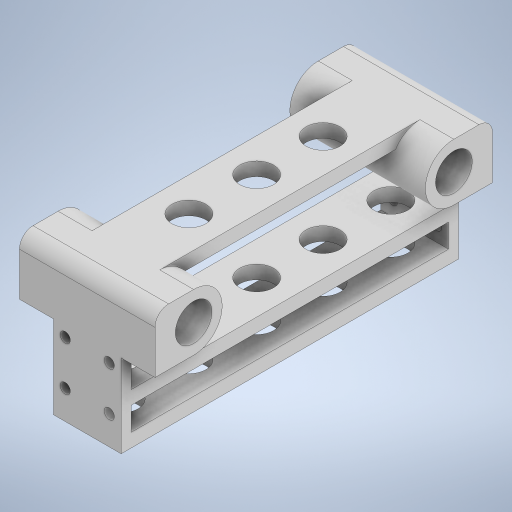
# Autodesk Inventor part: top
Saved by Autodesk Inventor 2024 (Build 280153000, 153)
## iProperties
Created: 2024-07-02
Part Number: top
Material: 일반
Document SubType Name: Modeling
Designer: Gihyeok Na
Density: 1 g/cm^3
Appearance: 기본값
Author: Gihyeok Na
Autodesk Inventor part; units mm, degrees
ref_plane "YZ Plane" through (0, 0, 0) normal (1, 0, 0) x (0, 1, 0)
ref_plane "XZ Plane" through (0, 0, 0) normal (0, 1, 0) x (-1, 0, 0)
ref_plane "XY Plane" through (0, 0, 0) normal (0, 0, 1) x (1, 0, 0)
sketch "스케치1" plane through (0, 0, 0) normal (1, 0, 0) x (0, 1, 0)
  line L0 (-15, -8.4) -> (15, -8.4)
  line L1 (15, -8.4) -> (15, -11.4)
  line L2 (15, -11.4) -> (-15, -11.4)
  line L3 (-15, -11.4) -> (-15, -8.4)
  line L4 (-15, -8.4) -> (15, -11.4) construction
  line L5 (15, -8.4) -> (-15, -11.4) construction
  line L6 (-10.7716, 0) -> (20.6854, 0) construction
  circle A0 centre (17.9, 0) radius 5.4
  circle A1 centre (17.9, 0) radius 8.4
  line L7 (9.5, -4.3302) -> (9.5, -23.7251) construction
  line L8 (15, -8.4) -> (17.9, -8.4)
  line L9 (9.5, 0) -> (9.5, -8.4)
  line L10 (56.0253, 38.4) -> (-49.003, 38.4) construction
  line L11 (-15, 85.2) -> (15, 85.2)
  line L12 (15, 85.2) -> (15, 88.2)
  line L13 (15, 88.2) -> (-15, 88.2)
  line L14 (-15, 88.2) -> (-15, 85.2)
  line L15 (-15, 85.2) -> (15, 88.2) construction
  line L16 (15, 85.2) -> (-15, 88.2) construction
  line L17 (-10.7716, 76.8) -> (20.6854, 76.8) construction
  circle A2 centre (17.9, 76.8) radius 5.4
  circle A3 centre (17.9, 76.8) radius 8.4
  line L18 (9.5, 81.1302) -> (9.5, 100.5251) construction
  line L19 (15, 85.2) -> (17.9, 85.2)
  line L20 (9.5, 76.8) -> (9.5, 85.2)
  line L21 (15, -11.4) -> (26.3, -11.4)
  line L22 (26.3, -11.4) -> (26.3, 0)
  line L23 (15, 88.2) -> (26.3, 88.2)
  line L24 (26.3, 88.2) -> (26.3, 76.8)
  point P0 (0, -9.9)
  point P1 (6.5, -8.4)
  point P2 (22.1201, -7.263)
  point P3 (0, 86.7)
  point P4 (6.5, 85.2)
  point P5 (22.1201, 84.063)
  dimension "d2" = 30
  dimension "d3" = 3
  dimension "d9" = 10.8
  dimension "d10" = 16.8
  dimension "d11" = 8.5
  dimension "d12" = 3
  dimension "d20" = 38.4
  constraints: 50 end point, 18 symmetric about line, 11 point on line, 7 point on circle, 4 centre point, 4 horizontal, 4 midpoint, 3 tangent, 2 coincident, 2 parallel, 1 perpendicular, 1 vertical, 2 other
  measures "d2" distance of L0.start L0.end
  measures "d3" distance of L0.end L1.end
  measures "d9" diameter of A0
  measures "d10" diameter of A1
  measures "d11" distance from line of point (6.5, -8.4) L1
  measures "d12" distance from line of L7 point (6.5, -8.4)
  measures "d20" distance from line of L10 A0.centre
extrude "돌출1" add sketch "스케치1" along normal mid plane 20
fillet "모깎기1" radius 4 2 edges at (0, 26.3, -11.4) (0, 26.3, 88.2)
sketch "스케치4" plane through (10, -15, -11.4) normal (0, 0, -1) x (-1, 0, 0)
  line L0 (-6.6272, 15) -> (50.9826, 15) construction
  line L1 (10, 54.1091) -> (10, -11.8144) construction
  circle A0 centre (3.5, 8.5) radius 1.5
  line L2 (20, 0) -> (0, 0) projected
  line L3 (0, 0) -> (0, 37.3) projected
  circle A1 centre (16.5, 8.5) radius 1.5
  circle A2 centre (3.5, 21.5) radius 1.5
  circle A3 centre (16.5, 21.5) radius 1.5
  circle A4 centre (10, 32.9) radius 1.25
  line L4 (20, 41.3) -> (0, 41.3) projected
  point P0 (10, 15)
  dimension "d22" = 3
  dimension "d23" = 8.5
  dimension "d24" = 3.5
  dimension "d27" = 2.5
  dimension "d28" = 8.4
  constraints: 5 centre point, 4 end point, 3 symmetric about line, 1 horizontal, 1 point on line, 1 vertical, 3 other
  measures "d22" diameter of A0
  measures "d23" distance from line of L2 A0.centre
  measures "d24" distance from line of L3 A0.centre
  measures "d27" diameter of A4
  measures "d28" distance from line of A4.centre L4
extrude "돌출4" cut sketch "스케치4" against normal through all contours A0 | A1 | A2 | A3
sketch "스케치5" plane through (-10, 0, 0) normal (-1, 0, 0) x (0, 0, 1)
  circle A0 centre (0, 17.9) radius 5.4 projected
  arc A1 (-7.4, 26.3) -> (-11.4, 22.3) centre (-7.4, 22.3) ccw projected
  line L0 (-11.4, 22.3) -> (-11.4, -15) projected
  line L1 (-11.4, -15) -> (-8.4, -15) projected
  line L2 (-8.4, -15) -> (-8.4, 9.5) projected
  line L3 (-8.4, 9.5) -> (0, 9.5) projected
  arc A2 (0, 9.5) -> (0, 26.3) centre (0, 17.9) ccw projected
  line L4 (0, 26.3) -> (-7.4, 26.3) projected
  circle A3 centre (76.8, 17.9) radius 5.4 projected
  arc A4 (88.2, 22.3) -> (84.2, 26.3) centre (84.2, 22.3) ccw projected
  line L5 (84.2, 26.3) -> (76.8, 26.3) projected
  arc A5 (76.8, 26.3) -> (76.8, 9.5) centre (76.8, 17.9) ccw projected
  line L6 (76.8, 9.5) -> (85.2, 9.5) projected
  line L7 (85.2, 9.5) -> (85.2, -15) projected
  line L8 (85.2, -15) -> (88.2, -15) projected
  line L9 (88.2, -15) -> (88.2, 22.3) projected
  line L10 (-8.4, -15) -> (85.2, -15)
  line L11 (-8.4, -11) -> (85.2, -11)
  line L12 (85.2, -15) -> (88.2, -15) projected
  line L13 (-8.4, 9.5) -> (-8.4, -15) projected
  line L14 (0, 26.3) -> (76.8, 26.3)
  circle A6 centre (0, 17.9) radius 5.4 projected
  circle A7 centre (76.8, 17.9) radius 5.4 projected
  line L15 (-8.4, -2.062) -> (85.2, -2.062) construction
  line L16 (-8.4, -4.062) -> (85.2, -4.062)
  line L17 (7.1554, 22.3) -> (69.6446, 22.3)
  line L18 (-8.4, -0.062) -> (85.2, -0.062)
  point P0 (0, 0)
  point P1 (0, -6.5)
  point P2 (0, 6.5)
  point P3 (0, 0)
  dimension "d29" = 4
  dimension "d31" = 8.5
  dimension "d32" = 13
  dimension "d33" = 6.5
  dimension "d34" = 2
  dimension "d35" = 4
  constraints: 14 end point, 6 point on line, 3 horizontal, 3 perpendicular, 2 point on circle, 2 symmetric about line, 2 tangent, 1 collinear
  measures "d29" distance between parallel lines of L10 L11
  measures "d31" distance from line of L10 point (0, -6.5)
  measures "d32" distance of point (0, -6.5) point (0, 6.5)
  measures "d33" distance of point (0, -6.5) point (0, 0)
  measures "d34" distance between parallel lines of L16 L15
  measures "d35" distance between parallel lines of L17 L14
extrude "돌출5" add sketch "스케치5" against normal up to surface (20 mm away) contours L14 A5 L17 A2 | L2 L11 L7 L10 | L2 L18 L7 L16
sketch "스케치6" plane through (-10, -15, -11.4) normal (0, -1, 0) x (1, 0, 0)
  circle A0 centre (10, 10) radius 5
  line L0 (0, 0) -> (20, 0) projected
  line L1 (10, 10) -> (10, 54.4458) construction
  circle A1 centre (10, 89.6) radius 5
  line L2 (0, 99.6) -> (20, 99.6) projected
  circle A2 centre (10, 30) radius 5
  circle A3 centre (10, 69.6) radius 5
  circle A4 centre (10, 49.6) radius 5
  point P0 (10, 11.4)
  dimension "d38" = 10
  dimension "d39" = 10
  dimension "d40" = 10
  dimension "d41" = 10
  dimension "d44" = 20
  dimension "d51" = 20
  constraints: 5 centre point, 3 vertical, 2 end point, 6 other
  measures "d38" diameter of A0
  measures "d39" distance from line of L1.start L0
  measures "d40" diameter of A1
  measures "d41" distance from line of L2 A1.centre
  measures "d44" distance of L1.start A2.centre
  measures "d51" distance of A1.centre A3.centre
extrude "돌출6" cut sketch "스케치6" against normal up to surface (14.938 mm away)
extrude "돌출7" cut sketch "스케치6" against normal through all contours A2 | A3 | A4
sketch "스케치7" plane through (-10, 0, 0) normal (-1, 0, 0) x (0, 0, 1)
  arc A0 (0, 9.5) -> (7.1554, 22.3) centre (0, 17.9) ccw projected
  arc A1 (69.6446, 22.3) -> (76.8, 9.5) centre (76.8, 17.9) ccw projected
  line L0 (-8.4, 9.5) -> (0, 9.5) projected
  line L1 (-11.4, 22.3) -> (-11.4, -15) projected
  arc A2 (-7.4, 26.3) -> (-11.4, 22.3) centre (-7.4, 22.3) ccw projected
  line L2 (84.2, 26.3) -> (-7.4, 26.3) projected
  arc A3 (88.2, 22.3) -> (84.2, 26.3) centre (84.2, 22.3) ccw projected
  line L3 (88.2, -15) -> (88.2, 22.3) projected
  line L4 (76.8, 9.5) -> (85.2, 9.5) projected
  line L5 (-8.4, 9.5) -> (-11.4, 9.5)
  line L6 (85.2, 9.5) -> (88.2, 9.5)
  arc A4 (7.1554, 22.3) -> (0, 26.3) centre (0, 17.9) ccw
  line L7 (7.1554, 22.3) -> (69.6446, 22.3) projected
  arc A5 (76.8, 26.3) -> (69.6446, 22.3) centre (76.8, 17.9) ccw
  circle A6 centre (0, 17.9) radius 5.4 projected
  circle A7 centre (76.8, 17.9) radius 5.4 projected
  point P0 (0, 0)
  constraints: 5 point on line, 4 end point, 4 point on circle, 2 centre point, 2 coincident, 1 horizontal
extrude "돌출8" add sketch "스케치7" along normal blind 10 contours L0 L5 L1 A2 L2 A4 A0 | A5 L2 A3 L3 L6 L4 A1
sketch "스케치8" plane through (10, 0, 0) normal (1, 0, 0) x (0, 0, -1)
  line L0 (0, 9.5) -> (8.4, 9.5) projected
  arc A0 (-7.1554, 22.3) -> (0, 9.5) centre (0, 17.9) ccw projected
  arc A1 (0, 26.3) -> (-7.1554, 22.3) centre (0, 17.9) ccw projected
  line L1 (7.4, 26.3) -> (-84.2, 26.3) projected
  arc A2 (11.4, 22.3) -> (7.4, 26.3) centre (7.4, 22.3) ccw projected
  line L2 (11.4, -15) -> (11.4, 22.3) projected
  circle A3 centre (0, 17.9) radius 5.4 projected
  line L3 (8.4, 9.5) -> (11.4, 9.5) projected
  arc A4 (-76.8, 9.5) -> (-69.6446, 22.3) centre (-76.8, 17.9) ccw projected
  line L4 (-85.2, 9.5) -> (-76.8, 9.5) projected
  arc A5 (-69.6446, 22.3) -> (-76.8, 26.3) centre (-76.8, 17.9) ccw projected
  arc A6 (-84.2, 26.3) -> (-88.2, 22.3) centre (-84.2, 22.3) ccw projected
  circle A7 centre (-76.8, 17.9) radius 5.4 projected
  line L5 (-88.2, 9.5) -> (-85.2, 9.5) projected
  line L6 (-88.2, 22.3) -> (-88.2, -15) projected
  point P0 (0, 0)
extrude "돌출9" add sketch "스케치8" along normal blind 10
sketch "스케치9" plane through (10, -15, -11.4) normal (0, 0, -1) x (-1, 0, 0)
  circle A0 centre (16.5, 8.5) radius 1.5 projected
  circle A1 centre (3.5, 8.5) radius 1.5 projected
  circle A2 centre (3.5, 21.5) radius 1.5 projected
  circle A3 centre (16.5, 21.5) radius 1.5 projected
  line L0 (-10, 37.3) -> (30, 37.3) projected
  line L1 (-10, 24.5) -> (-10, 37.3) projected
  line L2 (0, 24.5) -> (-10, 24.5) projected
  line L3 (0, 0) -> (0, 24.5) projected
  line L4 (20, 0) -> (0, 0) projected
  line L5 (20, 24.5) -> (20, 0) projected
  line L6 (20, 24.5) -> (30, 24.5) projected
  line L7 (30, 37.3) -> (30, 24.5) projected
  line L8 (5, 37.3) -> (5, 41.3) projected
  line L9 (5, 37.3) -> (5, 41.3) projected
  line L10 (5, 37.3) -> (5, 41.3) projected
  line L11 (30, 41.3) -> (-10, 41.3) projected
  line L12 (-10, 37.3) -> (30, 37.3) projected
  line L13 (30, 41.3) -> (30, 37.3) projected
  line L14 (30, 41.3) -> (-10, 41.3) projected
  line L15 (-10, 37.3) -> (-10, 41.3) projected
  line L16 (-10, 32.9) -> (30, 32.9) construction
  circle A4 centre (-5, 32.9) radius 1.25
  circle A5 centre (25, 32.9) radius 1.25
  point P0 (10, 15)
  dimension "d64" = 8.4
  dimension "d65" = 2.5
  dimension "d66" = 2.5
  dimension "d67" = 5
  dimension "d68" = 5
  constraints: 4 point on line, 2 centre point, 2 end point, 1 perpendicular
  measures "d64" distance between parallel lines of L16 L11
  measures "d65" diameter of A4
  measures "d66" diameter of A5
  measures "d67" distance from line of L1 A4.centre
  measures "d68" distance from line of A5.centre L7
